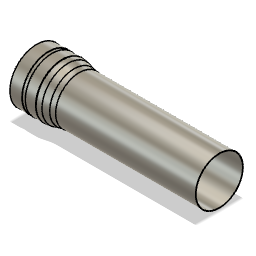
butted insulation tube v2 (Autodesk Fusion 360 design; units mm, degrees)
Autodesk Fusion 360 part; units mm, degrees
sketch "Sketch1" plane through (0, 0, 0) normal (0, 0, 1) x (1, 0, 0)
  line L0 (0, 40) -> (0, 37)
  line L1 (0, 37) -> (38, 37)
  line L2 (38, 37) -> (38, 39.5)
  line L3 (0, 40) -> (18, 40)
  line L4 (18, 40) -> (18, 39.5)
  line L5 (18, 39.5) -> (43, 39.5)
  line L6 (43, 39.5) -> (59.7942, 35)
  line L7 (59.7942, 35) -> (273, 35)
  line L8 (18, 40) -> (43.0658, 40)
  line L9 (43.0658, 40) -> (59.8601, 35.5)
  line L10 (59.8601, 35.5) -> (273, 35.5)
  line L11 (273, 35.5) -> (273, 35)
  line L12 (23, 40) -> (23, 39.5)
  dimension "d1" = -0.5
  dimension "d2" = 40
  dimension "d3" = 3
  dimension "d4" = 38
  dimension "d5" = 15
  dimension "d6" = 5
  dimension "d7" = 250
  dimension "d8" = 15
  dimension "d9" = 20
  dimension "d10" = 35
  constraint vertical L0
  constraint perpendicular L1 L2
  constraint perpendicular L0 L3
  constraint perpendicular L3 L4
  constraint perpendicular L4 L5
  constraint parallel L5 L7
  constraint perpendicular L7 L11
  constraint coincident L2.end L5
  constraint horizontal L8
  constraint collinear L3 L8
  constraint coincident L8 L12.start
  constraint coincident L5 L12.end
  constraint perpendicular L5 L12
  constraint coincident origin L0
  measures "d2" distance of origin L3
  measures "d3" distance of L1 L3
  measures "d4" distance of L0.end L1.end
  measures "d5" distance of L2 L12
  measures "d6" distance of L4 L12
  measures "d7" distance of L11 L12
  measures "d8" angle of L6 L7
  measures "d9" distance of L5.end L12.end
  measures "d10" distance of origin L7
revolve "Revolve1" add sketch "Sketch1" angle 360 about axis through (1.75, 0, 0) along (1, 0, 0) contours L0 L1 L2 L3 L4 L5 makes body 1
revolve "Revolve2" add sketch "Sketch1" angle 360 about axis through (1.75, 0, 0) along (1, 0, 0) separate body contours L5 L6 L7 L8 L9 L10 L11 L12 makes body 2
fillet "Fillet1" radius 30 4 edges at (59.8601, -12.8373, 33.0976) (43.0658, -14.4646, 37.2931) (59.7942, -12.6565, 32.6315) (43, -14.2838, 36.8269) on bodies 2
named bodies: "attachment tube", "insulation tube"
